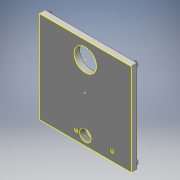
# Autodesk Inventor part: Moving Surface
Saved by Autodesk Inventor 2016 (Build 200138000, 138)
## iProperties
Created: 2016-02-22
Part Number: Moving Surface
Material: Generic
Document SubType Name: Modeling
Designer: Kenneth Daniel
Density: 1 g/cm^3
Appearance: Default
Author: Kenneth Daniel
Autodesk Inventor part; units mm, degrees
ref_plane "YZ Plane" through (0, 0, 0) normal (1, 0, 0) x (0, 1, 0)
ref_plane "XZ Plane" through (0, 0, 0) normal (0, 1, 0) x (-1, 0, 0)
ref_plane "XY Plane" through (0, 0, 0) normal (0, 0, 1) x (1, 0, 0)
sketch "Sketch1" plane through (0, 0, 0) normal (0, 1, 0) x (-1, 0, 0)
  line L0 (-40, 40) -> (-40, -40)
  line L1 (-40, -40) -> (40, -40)
  line L2 (40, -40) -> (40, 40)
  line L3 (40, 40) -> (-40, 40)
  line L4 (-40, 40) -> (40, -40) construction
  line L5 (-40, -40) -> (40, 40) construction
  point P0 (0, 0)
  dimension "d0" = 80
  dimension "d1" = 80
  constraints: 12 end point, 2 midpoint, 2 parallel, 1 perpendicular, 1 vertical
  measures "d0" distance of L0.start L0.end
  measures "d1" distance of L1.end L0.end
extrude "Extrusion1" add sketch "Sketch1" along normal blind 5
sketch "Sketch2" plane through (0, 5, 0) normal (0, 1, 0) x (1, 0, 0)
  circle A0 centre (0, -25) radius 9.75
  circle A1 centre (0, 32.0464) radius 5
  line L0 (40, 40) -> (-40, 40) construction
  line L1 (0, 40) -> (0, 0) construction
  line L2 (0, 0) -> (40, 40) construction
  line L3 (0, 0) -> (-40, 40) construction
  circle A2 centre (-8, 32.0464) radius 1.5
  line L4 (40, -40) -> (40, 40) projected
  line L5 (-8, 32.0464) -> (40, 32.0464) construction
  circle A3 centre (23.2847, 32.0464) radius 1.5
  dimension "d4" = 19.5
  dimension "d5" = 25
  dimension "d6" = 10
  dimension "d7" = 3
  dimension "d8" = 40
  dimension "d9" = 8
  dimension "d10" = 3
  constraints: 8 end point, 4 centre point, 2 point on line, 1 midpoint, 1 perpendicular, 1 vertical
  measures "d4" diameter of A0
  measures "d5" distance of L1.end A0.centre
  measures "d6" diameter of A1
  measures "d7" diameter of A2
  measures "d8" distance from line of L4 A1.centre
  measures "d9" distance of A1.centre L5.start
  measures "d10" diameter of A3
extrude "Extrusion2" cut sketch "Sketch2" against normal blind 5
sketch "Sketch3" plane through (0, 5, 0) normal (0, 1, 0) x (1, 0, 0)
  line L0 (-40, 40) -> (-40, -40) construction
  line L1 (40, 40) -> (-40, 40) construction
  line L2 (-40, -40) -> (40, 40) construction
  line L3 (-40, -40) -> (40, -40) construction
  line L4 (-40, 40) -> (40, -40) construction
  line L5 (-37, -40) -> (-37, 40) construction
  line L6 (-37, -37) -> (37, -37) construction
  line L7 (37, -37) -> (37, 37) construction
  line L8 (37, 37) -> (-37, 37) construction
  line L9 (-35.25, -38) -> (-35.25, -36)
  line L10 (-35.25, -36) -> (-38.75, -36)
  line L11 (-38.75, -36) -> (-38.75, -38)
  line L12 (-38.75, -38) -> (-35.25, -38)
  line L13 (-35.25, -38) -> (-38.75, -36) construction
  line L14 (-35.25, -36) -> (-38.75, -38) construction
  line L15 (-35.25, 36) -> (-35.25, 38)
  line L16 (-35.25, 38) -> (-38.75, 38)
  line L17 (-38.75, 38) -> (-38.75, 36)
  line L18 (-38.75, 36) -> (-35.25, 36)
  line L19 (-35.25, 36) -> (-38.75, 38) construction
  line L20 (-35.25, 38) -> (-38.75, 36) construction
  line L21 (35.25, 38) -> (35.25, 36)
  line L22 (35.25, 36) -> (38.75, 36)
  line L23 (38.75, 36) -> (38.75, 38)
  line L24 (38.75, 38) -> (35.25, 38)
  line L25 (35.25, 38) -> (38.75, 36) construction
  line L26 (35.25, 36) -> (38.75, 38) construction
  line L27 (35.25, -38) -> (35.25, -36)
  line L28 (35.25, -36) -> (38.75, -36)
  line L29 (38.75, -36) -> (38.75, -38)
  line L30 (38.75, -38) -> (35.25, -38)
  line L31 (35.25, -38) -> (38.75, -36) construction
  line L32 (35.25, -36) -> (38.75, -38) construction
  point P0 (0, 0)
  dimension "d13" = 3
  dimension "d14" = 2
  dimension "d15" = 3.5
  dimension "d16" = 2
  dimension "d17" = 3.5
  dimension "d18" = 3.5
  constraints: 60 end point, 8 midpoint, 8 parallel, 8 point on line, 7 perpendicular
  measures "d13" distance between parallel lines of L5 L0
  measures "d14" distance of L9.start L9.end
  measures "d15" distance of L10.end L9.end
  measures "d16" distance of L15.start L15.end
  measures "d17" distance of L16.end L15.end
  measures "d18" distance of L22.end L21.end
extrude "Extrusion3" add sketch "Sketch3" along normal blind 3.5
full round fillet "Fillet1" first side at (-35.25, 6.1667, 37.3333) centre faces at (-36.4167, 8.5, 37.3333) second side at (-38.75, 6.1667, 36.6667)
full round fillet "Fillet2" first side at (-38.75, 6.1667, -37.3333) centre faces at (-36.4167, 8.5, -36.6667) second side at (-35.25, 6.1667, -36.6667)
full round fillet "Fillet3" first side at (38.75, 6.1667, -36.6667) centre faces at (36.4167, 8.5, -37.3333) second side at (35.25, 6.1667, -37.3333)
full round fillet "Fillet4" first side at (35.25, 6.1667, 37.3333) centre faces at (36.4167, 8.5, 36.6667) second side at (38.75, 6.1667, 36.6667)
sketch "Sketch4" plane through (-38.75, 5, 38) normal (0, 0, 1) x (1, 0, 0)
  arc A0 (3.5, 1.75) -> (0, 1.75) centre (1.75, 1.75) ccw projected
  circle A1 centre (1.75, 1.75) radius 1
  arc A2 (77.5, 1.75) -> (74, 1.75) centre (75.75, 1.75) ccw projected
  circle A3 centre (75.75, 1.75) radius 1
  point P0 (38.75, -5)
  dimension "d21" = 2
  constraints: 2 centre point, 2 coincident
  measures "d21" diameter of A1
extrude "Extrusion4" cut sketch "Sketch4" against normal up to surface (76 mm away)
sketch "Sketch5" plane through (0, 0, 0) normal (0, -1, 0) x (1, 0, 0)
  circle A0 centre (0, -32.0464) radius 5 projected
  circle A1 centre (-8, -32.0464) radius 1.5 projected
  circle A2 centre (23.2847, -32.0464) radius 1.5 projected
  circle A3 centre (0, 25) radius 9.75 projected
  line L0 (40, 40) -> (40, -40) projected
  line L1 (-40, 40) -> (40, 40) projected
  line L2 (-40, -40) -> (-40, 40) projected
  line L3 (40, -40) -> (-40, -40) projected
  point P0 (0, 0)
body "Solid1"
